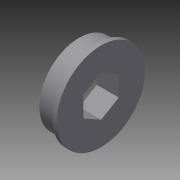
# Autodesk Inventor part: hexagon bearing
Saved by Autodesk Inventor 2015 (Build 190159000, 159)
## iProperties
Created: 2015-01-17
Part Number: hexagon bearing
Material: Generic
Document SubType Name: Modeling
Designer: whitaus15
Density: 1 g/cm^3
Appearance: Default
Author: whitaus15
Autodesk Inventor part; units mm, degrees
ref_plane "YZ Plane" through (0, 0, 0) normal (1, 0, 0) x (0, 1, 0)
ref_plane "XZ Plane" through (0, 0, 0) normal (0, 1, 0) x (-1, 0, 0)
ref_plane "XY Plane" through (0, 0, 0) normal (0, 0, 1) x (1, 0, 0)
sketch "Sketch1" plane through (0, 0, 0) normal (1, 0, 0) x (0, 1, 0)
  circle A0 centre (0, 0) radius 14.2875
  dimension "d0" = 28.575
  constraints: 1 centre point, 1 coincident
  measures "d0" diameter of A0
extrude "Extrusion1" add sketch "Sketch1" along normal blind 7.9248
sketch "Sketch4" plane through (7.9248, 0, 0) normal (1, 0, 0) x (0, 0, -1)
  line L0 (6.2959, 3.7584) -> (6.4028, -3.5732)
  line L1 (6.4028, -3.5732) -> (0.1069, -7.3316)
  line L2 (0.1069, -7.3316) -> (-6.2959, -3.7584)
  line L3 (-6.2959, -3.7584) -> (-6.4028, 3.5732)
  line L4 (-6.4028, 3.5732) -> (-0.1069, 7.3316)
  line L5 (-0.1069, 7.3316) -> (6.2959, 3.7584)
  point P0 (0, 0)
  point P1 (0, 0)
  dimension "d16" = 12.7
  constraints: 12 end point, 1 coincident, 13 other
  measures "d16" distance between parallel lines of L2 L5
extrude "Extrusion2" cut sketch "Sketch4" against normal blind 279.4
sketch "Sketch5" plane through (7.9248, 0, 0) normal (1, 0, 0) x (0, 0, -1)
  circle A0 centre (0, 0) radius 15.875
  dimension "d7" = 31.75
  constraints: 1 centre point, 1 coincident
  measures "d7" diameter of A0
extrude "Extrusion3" add sketch "Sketch5" against normal blind 1.6002
extrude "Extrusion4" cut sketch "Sketch4" against normal blind 1.6002
extrude "Extrusion5" add sketch "Sketch4" against normal blind 2.54
extrude "Extrusion6" cut sketch "Sketch4" against normal blind 2.54
body "Solid1"
